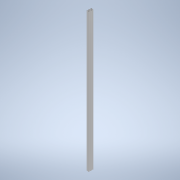
# Autodesk Inventor part: 40-4080-25-CL
Saved by Autodesk Inventor 2021 (Build 250183000, 183)
## iProperties
Category: PARTsolutions
Company: 8020
Part Number: 40-4080-25-CL
Material: Aluminum 6061
Catalog Web Link: www.cadenas.de
Description: 40-4080, 40-4080-Black-T-Slotted Profile - 40 Series
Vendor: 8020
Document SubType Name: Modeling
Designer: partserver
Manufacturer: 8020
Mass: 104.745 g
Surface Area: 180.679 cm^2
Volume: 38.7945 cm^3
Density: 2.7 g/cm^3
Appearance: Aluminum - Flat
PSOL_IDENT_0: {$CADENAS_DATA\23d-libs\8020\metric\profiles\40_series\40_4080.prj},191 {VTYP=3D},{NB=40-4080-25-CL}
PSOL_IDENT_1: ,{LINA=40-4080-25},{NN=40-4080, 40-4080-Black},{DATE=31.07.2020 09:21:33},{GEOMDATE=05.11.2018 21:41
PSOL_IDENT_2: :00},{VERSION=},{LINEID=10},{WBVAR=FINISH,LS,L},{WBNUMERIC=L}  {NB=40-4080-25-CL},{LINA=40-4080-25},
PSOL_IDENT_3: {KT=DUMMY},{PN=40-4080-25},{PN1=40-4080},{SERIES=40-4080},{MAT=6105-T5 Aluminum},{FINISH=CA},{LS=-CL
PSOL_IDENT_4: },{L=25.00},{W=4.1528},{LALG=[25:6000/0.05]},{MIX=97.6618},{MIY=25.2917},{EA=15.4345},{CLR=.75,.75,.
PSOL_IDENT_5: 75},{FIN=Clear Anodize}
NB: 40-4080-25-CL
NN: 40-4080, 40-4080-Black
NT: T-Slotted Profile - 40 Series
NBSYN: $PN.$LS.
LINA: 40-4080-25
CATALOG: 80/20
PN: 40-4080-25
SERIES: 40-4080
MAT: 6105-T5 Aluminum
FINISH: Clear Anodize
LS: Custom Length
L: 25
W: 4.1528
MIX: 97.6618
MIY: 25.2917
EA: 15.4345
FIN: Clear Anodize
SUPPLIER: 8020
ARTICLENO: 40-4080-25-CL
BOMINFO: 40-4080-25
CREATOR: CADENAS GmbH
Title: 40-4080-25
Author: Cadenas PARTsolutions
Comments: T-Slotted Profile - 40 Series
Autodesk Inventor part; units mm, degrees
ref_plane "YZ Plane" through (0, 0, 0) normal (1, 0, 0) x (0, 1, 0)
ref_plane "XZ Plane" through (0, 0, 0) normal (0, 1, 0) x (-1, 0, 0)
ref_plane "XY Plane" through (0, 0, 0) normal (0, 0, 1) x (1, 0, 0)
sketch "Sketch_1" plane through (0, 0, 0) normal (0, 0, 1) x (1, 0, 0)
  line L0 (-20, 56.83) -> (-20, 45.6904)
  arc A0 (-20, 45.6904) -> (-18.43, 44.1204) centre (-18.43, 45.6904) ccw
  line L1 (-18.43, 44.1204) -> (-17.25, 44.1204)
  arc A1 (-17.25, 44.1204) -> (-15.68, 45.6904) centre (-17.25, 45.6904) ccw
  line L2 (-15.68, 45.6904) -> (-15.68, 48.7154)
  arc A2 (-14.11, 50.2854) -> (-15.68, 48.7154) centre (-14.11, 48.7154) ccw
  line L3 (-14.11, 50.2854) -> (-13.6549, 50.2854)
  arc A3 (-13.1175, 50.0628) -> (-13.6549, 50.2854) centre (-13.6549, 49.5254) ccw
  line L4 (-13.1175, 50.0628) -> (-9.1098, 46.0551)
  arc A4 (-7.685, 42.6153) -> (-9.1098, 46.0551) centre (-12.5496, 42.6153) ccw
  line L5 (-7.685, 42.6153) -> (-7.685, 37.3847)
  arc A5 (-9.1098, 33.9449) -> (-7.685, 37.3847) centre (-12.5496, 37.3847) ccw
  line L6 (-9.1098, 33.9449) -> (-13.1175, 29.9372)
  arc A6 (-13.6549, 29.7146) -> (-13.1175, 29.9372) centre (-13.6549, 30.4746) ccw
  line L7 (-13.6549, 29.7146) -> (-14.11, 29.7146)
  arc A7 (-15.68, 31.2846) -> (-14.11, 29.7146) centre (-14.11, 31.2846) ccw
  line L8 (-15.68, 31.2846) -> (-15.68, 34.3096)
  arc A8 (-15.68, 34.3096) -> (-17.25, 35.8796) centre (-17.25, 34.3096) ccw
  line L9 (-17.25, 35.8796) -> (-18.43, 35.8796)
  arc A9 (-18.43, 35.8796) -> (-20, 34.3096) centre (-18.43, 34.3096) ccw
  line L10 (-20, 34.3096) -> (-20, 5.6904)
  arc A10 (-20, 5.6904) -> (-18.43, 4.1204) centre (-18.43, 5.6904) ccw
  line L11 (-18.43, 4.1204) -> (-17.25, 4.1204)
  arc A11 (-17.25, 4.1204) -> (-15.68, 5.6904) centre (-17.25, 5.6904) ccw
  line L12 (-15.68, 5.6904) -> (-15.68, 8.7154)
  arc A12 (-14.11, 10.2854) -> (-15.68, 8.7154) centre (-14.11, 8.7154) ccw
  line L13 (-14.11, 10.2854) -> (-13.6549, 10.2854)
  arc A13 (-13.1175, 10.0628) -> (-13.6549, 10.2854) centre (-13.6549, 9.5254) ccw
  line L14 (-13.1175, 10.0628) -> (-9.1098, 6.0551)
  arc A14 (-7.685, 2.6153) -> (-9.1098, 6.0551) centre (-12.5496, 2.6153) ccw
  line L15 (-7.685, 2.6153) -> (-7.685, -2.6153)
  arc A15 (-9.1098, -6.0551) -> (-7.685, -2.6153) centre (-12.5496, -2.6153) ccw
  line L16 (-9.1098, -6.0551) -> (-13.1175, -10.0628)
  arc A16 (-13.6549, -10.2854) -> (-13.1175, -10.0628) centre (-13.6549, -9.5254) ccw
  line L17 (-13.6549, -10.2854) -> (-14.11, -10.2854)
  arc A17 (-15.68, -8.7154) -> (-14.11, -10.2854) centre (-14.11, -8.7154) ccw
  line L18 (-15.68, -8.7154) -> (-15.68, -5.6904)
  arc A18 (-15.68, -5.6904) -> (-17.25, -4.1204) centre (-17.25, -5.6904) ccw
  line L19 (-17.25, -4.1204) -> (-18.43, -4.1204)
  arc A19 (-18.43, -4.1204) -> (-20, -5.6904) centre (-18.43, -5.6904) ccw
  line L20 (-20, -5.6904) -> (-20, -16.83)
  arc A20 (-20, -16.83) -> (-16.83, -20) centre (-16.83, -16.83) ccw
  line L21 (-16.83, -20) -> (-5.6904, -20)
  arc A21 (-5.6904, -20) -> (-4.1204, -18.43) centre (-5.6904, -18.43) ccw
  line L22 (-4.1204, -18.43) -> (-4.1204, -17.25)
  arc A22 (-4.1204, -17.25) -> (-5.6904, -15.68) centre (-5.6904, -17.25) ccw
  line L23 (-5.6904, -15.68) -> (-8.7154, -15.68)
  arc A23 (-10.2854, -14.11) -> (-8.7154, -15.68) centre (-8.7154, -14.11) ccw
  line L24 (-10.2854, -14.11) -> (-10.2854, -13.6549)
  arc A24 (-10.0628, -13.1175) -> (-10.2854, -13.6549) centre (-9.5254, -13.6549) ccw
  line L25 (-10.0628, -13.1175) -> (-6.0551, -9.1098)
  arc A25 (-2.6153, -7.685) -> (-6.0551, -9.1098) centre (-2.6153, -12.5496) ccw
  line L26 (-2.6153, -7.685) -> (2.6153, -7.685)
  arc A26 (6.0551, -9.1098) -> (2.6153, -7.685) centre (2.6153, -12.5496) ccw
  line L27 (6.0551, -9.1098) -> (10.0628, -13.1175)
  arc A27 (10.2854, -13.6549) -> (10.0628, -13.1175) centre (9.5254, -13.6549) ccw
  line L28 (10.2854, -13.6549) -> (10.2854, -14.11)
  arc A28 (8.7154, -15.68) -> (10.2854, -14.11) centre (8.7154, -14.11) ccw
  line L29 (8.7154, -15.68) -> (5.6904, -15.68)
  arc A29 (5.6904, -15.68) -> (4.1204, -17.25) centre (5.6904, -17.25) ccw
  line L30 (4.1204, -17.25) -> (4.1204, -18.43)
  arc A30 (4.1204, -18.43) -> (5.6904, -20) centre (5.6904, -18.43) ccw
  line L31 (5.6904, -20) -> (16.83, -20)
  arc A31 (16.83, -20) -> (20, -16.83) centre (16.83, -16.83) ccw
  line L32 (20, -16.83) -> (20, -5.6904)
  arc A32 (20, -5.6904) -> (18.43, -4.1204) centre (18.43, -5.6904) ccw
  line L33 (18.43, -4.1204) -> (17.25, -4.1204)
  arc A33 (17.25, -4.1204) -> (15.68, -5.6904) centre (17.25, -5.6904) ccw
  line L34 (15.68, -5.6904) -> (15.68, -8.7154)
  arc A34 (14.11, -10.2854) -> (15.68, -8.7154) centre (14.11, -8.7154) ccw
  line L35 (14.11, -10.2854) -> (13.6549, -10.2854)
  arc A35 (13.1175, -10.0628) -> (13.6549, -10.2854) centre (13.6549, -9.5254) ccw
  line L36 (13.1175, -10.0628) -> (9.1098, -6.0551)
  arc A36 (7.685, -2.6153) -> (9.1098, -6.0551) centre (12.5496, -2.6153) ccw
  line L37 (7.685, -2.6153) -> (7.685, 2.6153)
  arc A37 (9.1098, 6.0551) -> (7.685, 2.6153) centre (12.5496, 2.6153) ccw
  line L38 (9.1098, 6.0551) -> (13.1175, 10.0628)
  arc A38 (13.6549, 10.2854) -> (13.1175, 10.0628) centre (13.6549, 9.5254) ccw
  line L39 (13.6549, 10.2854) -> (14.11, 10.2854)
  arc A39 (15.68, 8.7154) -> (14.11, 10.2854) centre (14.11, 8.7154) ccw
  line L40 (15.68, 8.7154) -> (15.68, 5.6904)
  arc A40 (15.68, 5.6904) -> (17.25, 4.1204) centre (17.25, 5.6904) ccw
  line L41 (17.25, 4.1204) -> (18.43, 4.1204)
  arc A41 (18.43, 4.1204) -> (20, 5.6904) centre (18.43, 5.6904) ccw
  line L42 (20, 5.6904) -> (20, 34.3096)
  arc A42 (20, 34.3096) -> (18.43, 35.8796) centre (18.43, 34.3096) ccw
  line L43 (18.43, 35.8796) -> (17.25, 35.8796)
  arc A43 (17.25, 35.8796) -> (15.68, 34.3096) centre (17.25, 34.3096) ccw
  line L44 (15.68, 34.3096) -> (15.68, 31.2846)
  arc A44 (14.11, 29.7146) -> (15.68, 31.2846) centre (14.11, 31.2846) ccw
  line L45 (14.11, 29.7146) -> (13.6549, 29.7146)
  arc A45 (13.1175, 29.9372) -> (13.6549, 29.7146) centre (13.6549, 30.4746) ccw
  line L46 (13.1175, 29.9372) -> (9.1098, 33.9449)
  arc A46 (7.685, 37.3847) -> (9.1098, 33.9449) centre (12.5496, 37.3847) ccw
  line L47 (7.685, 37.3847) -> (7.685, 42.6153)
  arc A47 (9.1098, 46.0551) -> (7.685, 42.6153) centre (12.5496, 42.6153) ccw
  line L48 (9.1098, 46.0551) -> (13.1175, 50.0628)
  arc A48 (13.6549, 50.2854) -> (13.1175, 50.0628) centre (13.6549, 49.5254) ccw
  line L49 (13.6549, 50.2854) -> (14.11, 50.2854)
  arc A49 (15.68, 48.7154) -> (14.11, 50.2854) centre (14.11, 48.7154) ccw
  line L50 (15.68, 48.7154) -> (15.68, 45.6904)
  arc A50 (15.68, 45.6904) -> (17.25, 44.1204) centre (17.25, 45.6904) ccw
  line L51 (17.25, 44.1204) -> (18.43, 44.1204)
  arc A51 (18.43, 44.1204) -> (20, 45.6904) centre (18.43, 45.6904) ccw
  line L52 (20, 45.6904) -> (20, 56.83)
  arc A52 (20, 56.83) -> (16.83, 60) centre (16.83, 56.83) ccw
  line L53 (16.83, 60) -> (5.6904, 60)
  arc A53 (5.6904, 60) -> (4.1204, 58.43) centre (5.6904, 58.43) ccw
  line L54 (4.1204, 58.43) -> (4.1204, 57.25)
  arc A54 (4.1204, 57.25) -> (5.6904, 55.68) centre (5.6904, 57.25) ccw
  line L55 (5.6904, 55.68) -> (8.7154, 55.68)
  arc A55 (10.2854, 54.11) -> (8.7154, 55.68) centre (8.7154, 54.11) ccw
  line L56 (10.2854, 54.11) -> (10.2854, 53.6549)
  arc A56 (10.0628, 53.1175) -> (10.2854, 53.6549) centre (9.5254, 53.6549) ccw
  line L57 (10.0628, 53.1175) -> (6.0551, 49.1098)
  arc A57 (2.6153, 47.685) -> (6.0551, 49.1098) centre (2.6153, 52.5496) ccw
  line L58 (2.6153, 47.685) -> (-2.6153, 47.685)
  arc A58 (-6.0551, 49.1098) -> (-2.6153, 47.685) centre (-2.6153, 52.5496) ccw
  line L59 (-6.0551, 49.1098) -> (-10.0628, 53.1175)
  arc A59 (-10.2854, 53.6549) -> (-10.0628, 53.1175) centre (-9.5254, 53.6549) ccw
  line L60 (-10.2854, 53.6549) -> (-10.2854, 54.11)
  arc A60 (-8.7154, 55.68) -> (-10.2854, 54.11) centre (-8.7154, 54.11) ccw
  line L61 (-8.7154, 55.68) -> (-5.6904, 55.68)
  arc A61 (-5.6904, 55.68) -> (-4.1204, 57.25) centre (-5.6904, 57.25) ccw
  line L62 (-4.1204, 57.25) -> (-4.1204, 58.43)
  arc A62 (-4.1204, 58.43) -> (-5.6904, 60) centre (-5.6904, 58.43) ccw
  line L63 (-5.6904, 60) -> (-16.83, 60)
  arc A63 (-16.83, 60) -> (-20, 56.83) centre (-16.83, 56.83) ccw
  circle A64 centre (0, 0) radius 3.405
  circle A65 centre (0, 40) radius 3.405
  arc A66 (-15.68, 15.9286) -> (-14.41, 14.6586) centre (-14.41, 15.9286) ccw
  line L64 (-14.41, 14.6586) -> (-12.13, 14.6586)
  arc A67 (-11.232, 14.2867) -> (-12.13, 14.6586) centre (-12.13, 13.3886) ccw
  line L65 (-11.232, 14.2867) -> (-6.0551, 9.1098)
  arc A68 (-6.0551, 9.1098) -> (-2.6153, 7.685) centre (-2.6153, 12.5496) ccw
  line L66 (-2.6153, 7.685) -> (2.6153, 7.685)
  arc A69 (2.6153, 7.685) -> (6.0551, 9.1098) centre (2.6153, 12.5496) ccw
  line L67 (6.0551, 9.1098) -> (11.232, 14.2867)
  arc A70 (12.13, 14.6586) -> (11.232, 14.2867) centre (12.13, 13.3886) ccw
  line L68 (12.13, 14.6586) -> (14.41, 14.6586)
  arc A71 (14.41, 14.6586) -> (15.68, 15.9286) centre (14.41, 15.9286) ccw
  line L69 (15.68, 15.9286) -> (15.68, 24.0714)
  arc A72 (15.68, 24.0714) -> (14.41, 25.3414) centre (14.41, 24.0714) ccw
  line L70 (14.41, 25.3414) -> (12.13, 25.3414)
  arc A73 (11.232, 25.7133) -> (12.13, 25.3414) centre (12.13, 26.6114) ccw
  line L71 (11.232, 25.7133) -> (6.0551, 30.8902)
  arc A74 (6.0551, 30.8902) -> (2.6153, 32.315) centre (2.6153, 27.4504) ccw
  line L72 (2.6153, 32.315) -> (-2.6153, 32.315)
  arc A75 (-2.6153, 32.315) -> (-6.0551, 30.8902) centre (-2.6153, 27.4504) ccw
  line L73 (-6.0551, 30.8902) -> (-11.232, 25.7133)
  arc A76 (-12.13, 25.3414) -> (-11.232, 25.7133) centre (-12.13, 26.6114) ccw
  line L74 (-12.13, 25.3414) -> (-14.41, 25.3414)
  arc A77 (-14.41, 25.3414) -> (-15.68, 24.0714) centre (-14.41, 24.0714) ccw
  line L75 (-15.68, 24.0714) -> (-15.68, 15.9286)
  constraints: 152 end point, 152 point on circle, 78 centre point
extrude "Extrusion1" add sketch "Sketch_1" against normal blind 25
ref_plane "1_XY" through (0, 0, 0) normal (0, 0, 1) x (1, 0, 0)
ref_plane "1_YZ" through (0, 0, 0) normal (1, 0, 0) x (0, 1, 0)
ref_plane "1_ZX" through (0, 0, 0) normal (0, 1, 0) x (0, 0, 1)
ref_plane "to_parts_XY" through (0, 20, -12.5) normal (0, 0, 1) x (1, 0, 0)
ref_plane "to_parts_YZ" through (0, 20, -12.5) normal (1, 0, 0) x (0, 1, 0)
ref_plane "to_parts_ZX" through (0, 20, -12.5) normal (0, 1, 0) x (0, 0, 1)
thicken "Thicken1" operation add thickness 0.4 both sides no extend neighbours yes toward (0, 0, -1) faces at (-18.56, 18.6429, -25)
thicken "Thicken2" operation add thickness 2413 both sides no extend neighbours yes toward (0, 0, -1) faces at (-18.56, 21.3571, -25.4)
body "Solid1"
